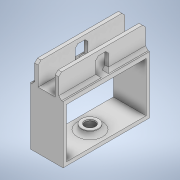
# Autodesk Inventor part: Koszyk_v2
Saved by Autodesk Inventor 2020 (Build 240168000, 168)
## iProperties
Created: 2020-03-14
Part Number: Koszyk_v2
Material: Generic
Document SubType Name: Modeling
Designer: atmat
Density: 1 g/cm^3
Appearance: Default
Author: atmat
Autodesk Inventor part; units mm, degrees
ref_plane "YZ Plane" through (0, 0, 0) normal (1, 0, 0) x (0, 1, 0)
ref_plane "XZ Plane" through (0, 0, 0) normal (0, 1, 0) x (-1, 0, 0)
ref_plane "XY Plane" through (0, 0, 0) normal (0, 0, 1) x (1, 0, 0)
sketch "Sketch1" plane through (0, 0, 0) normal (0, 1, 0) x (-1, 0, 0)
  line L0 (6, 30.5) -> (-6, 30.5)
  line L1 (-6, 30.5) -> (-6, -30.5)
  line L2 (-6, -30.5) -> (6, -30.5)
  line L3 (6, -30.5) -> (6, 30.5)
  line L4 (8.5, 30.5) -> (-8.5, 30.5)
  line L5 (-8.5, 30.5) -> (-8.5, -30.5)
  line L6 (-8.5, -30.5) -> (8.5, -30.5)
  line L7 (8.5, -30.5) -> (8.5, 30.5)
  point P0 (0, 0)
  point P1 (-6, 30.5)
  dimension "d0" = 61
  dimension "d1" = 30.5
  dimension "d2" = 0
  dimension "d3" = 0
  dimension "d4" = 2.5
  dimension "d5" = 2.5
  dimension "d6" = 12
  dimension "d7" = 6
  constraints: 16 end point, 4 parallel, 2 horizontal, 2 perpendicular
  measures "d0" distance of L6.end L4.start
  measures "d1" distance from line of point (0, 0) L4
  measures "d2" distance between parallel lines of L4 L0
  measures "d3" distance between parallel lines of L6 L2
  measures "d4" distance between parallel lines of L7 L3
  measures "d5" distance between parallel lines of L5 L1
  measures "d6" distance between parallel lines of L3 L1
  measures "d7" distance from line of point (0, 0) L3
extrude "Extrusion1" add sketch "Sketch1" along normal blind 15.5 contours L4 L7 L6 L3 | L1 L6 L5 L4
sketch "Sketch2" plane through (0, 0, 0) normal (0, 1, 0) x (-1, 0, 0)
  line L0 (-11.5, 28) -> (11.5, 28)
  line L1 (11.5, 28) -> (11.5, -28)
  line L2 (11.5, -28) -> (-11.5, -28)
  line L3 (-11.5, -28) -> (-11.5, 28)
  line L4 (-8.5, 30.5) -> (-8.5, -30.5) projected
  line L5 (8.5, -30.5) -> (8.5, 30.5) projected
  point P0 (0, 0)
  dimension "d10" = 56
  dimension "d11" = 28
  dimension "d12" = 3
  dimension "d13" = 3
  constraints: 8 end point, 2 parallel, 1 horizontal, 1 perpendicular
  measures "d10" distance of L2.end L0.start
  measures "d11" distance from line of point (0, 0) L0
  measures "d12" distance between parallel lines of L4 L3
  measures "d13" distance between parallel lines of L5 L1
extrude "Extrusion2" add sketch "Sketch2" against normal blind 3
sketch "Sketch3" plane through (0, -3, 0) normal (0, -1, 0) x (1, 0, 0)
  line L0 (11.5, -30.5) -> (-11.5, -30.5)
  line L1 (-11.5, -30.5) -> (-11.5, 30.5)
  line L2 (-11.5, 30.5) -> (11.5, 30.5)
  line L3 (11.5, 30.5) -> (11.5, -30.5)
  line L4 (11.5, -28) -> (11.5, 28) projected
  line L5 (-11.5, 28) -> (-11.5, -28) projected
  line L6 (-11.5, -28) -> (11.5, -28) projected
  line L7 (11.5, 28) -> (-11.5, 28) projected
  point P0 (0, 0)
  point P1 (11.5, -28)
  point P2 (-11.5, -28)
  point P3 (-11.5, 28)
  point P4 (11.5, 28)
  dimension "d16" = 0
  dimension "d17" = 0
  dimension "d18" = 2.5
  dimension "d19" = 2.5
  constraints: 8 end point, 2 parallel, 1 horizontal, 1 perpendicular
  measures "d16" distance between parallel lines of L4 L3
  measures "d17" distance between parallel lines of L5 L1
  measures "d18" distance between parallel lines of L6 L0
  measures "d19" distance between parallel lines of L2 L7
extrude "Extrusion3" add sketch "Sketch3" along normal blind 35 and the other way blind 3 contours L0 L1 L6 L3 | L7 L1 L2 L3
sketch "Sketch4" plane through (0, -38, 0) normal (0, -1, 0) x (1, 0, 0)
  line L0 (11.5, 30.5) -> (11.5, -30.5) projected
  line L1 (-11.5, -30.5) -> (-11.5, 30.5) projected
  line L2 (11.5, -30.5) -> (-11.5, -30.5)
  line L3 (-11.5, -30.5) -> (-11.5, 30.5)
  line L4 (-11.5, 30.5) -> (11.5, 30.5)
  line L5 (11.5, 30.5) -> (11.5, -30.5)
  point P0 (0, 0)
  constraints: 8 end point, 2 parallel, 1 horizontal, 1 perpendicular
extrude "Extrusion4" add sketch "Sketch4" along normal blind 2.5
sketch "Sketch5" plane through (0, -40.5, 0) normal (0, -1, 0) x (1, 0, 0)
  circle A0 centre (0, 0) radius 6
  dimension "d26" = 12
  constraints: 1 centre point, 1 coincident
  measures "d26" diameter of A0
extrude "Extrusion5" add sketch "Sketch5" along normal blind 3 and the other way blind 6
sketch "Sketch6" plane through (0, -43.5, 0) normal (0, -1, 0) x (1, 0, 0)
  circle A0 centre (0, 0) radius 3.75
  circle A1 centre (0, 0) radius 5
  dimension "d31" = 7.5
  dimension "d32" = 10
  constraints: 2 centre point, 2 coincident
  measures "d31" diameter of A0
  measures "d32" diameter of A1
extrude "Extrusion6" cut sketch "Sketch6" against normal blind 8
sketch "Sketch7" plane through (0, 0, 0) normal (0, 1, 0) x (1, 0, 0)
  line L0 (-11.5, -4.5) -> (12.0053, -4.5)
  line L1 (12.0053, -4.5) -> (12.0053, 4.5)
  line L2 (12.0053, 4.5) -> (-11.5, 4.5)
  line L3 (-11.5, 4.5) -> (-11.5, -4.5)
  line L4 (-11.5, 28) -> (-11.5, -28) projected
  point P0 (0, 0)
  point P1 (-12, 31)
  point P2 (-12, -31)
  dimension "d35" = 0
  dimension "d36" = 9
  dimension "d37" = 4.5
  constraints: 8 end point, 2 parallel, 1 horizontal, 1 perpendicular, 1 other
  measures "d35" horizontal extent of L3
  measures "d36" distance between parallel lines of L2 L0
  measures "d37" distance from line of point (0, 0) L2
extrude "Extrusion7" cut sketch "Sketch7" along normal blind 12.5
chamfer "Chamfer1" distance 2 angle 45 12 edges at (-7.25, 12.5, 4.5) (-7.25, 0, 4.5) (7.25, 0, 4.5) (7.25, 12.5, -4.5) (7.25, 12.5, 4.5) (-7.25, 12.5, -4.5) (7.25, 0, -4.5) (-7.25, 0, -4.5) (8.5, 0, 17.5) (8.5, 0, -17.5) (-8.5, 0, -17.5) (-8.5, 0, 17.5)
chamfer "Chamfer2" distance 2 angle 45 4 edges at (-7.25, 15.5, 30.5) (7.25, 15.5, 30.5) (-7.25, 15.5, -30.5) (7.25, 15.5, -30.5)
fillet "Fillet1" radius 3 2 edges at (-6, -40.5, 0) (-6, -38, 0)
sketch "Sketch8" plane through (0, -43.5, 0) normal (0, -1, 0) x (1, 0, 0)
  circle A0 centre (0, 0) radius 3.75
  constraints: 1 centre point, 1 coincident
extrude "Extrusion8" cut sketch "Sketch8" against normal blind 10
body "Solid1"
